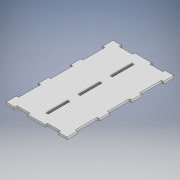
# Autodesk Inventor part: Lateral 1
Saved by Autodesk Inventor 2020 (Build 240168000, 168)
## iProperties
Created: 2020-03-11
Part Number: Lateral 1
Material: Generic
Document SubType Name: Modeling
Designer: José Javier Estrada
Density: 1 g/cm^3
Appearance: Default
Author: José Javier Estrada
Autodesk Inventor part; units mm, degrees
ref_plane "YZ Plane" through (0, 0, 0) normal (1, 0, 0) x (0, 1, 0)
ref_plane "XZ Plane" through (0, 0, 0) normal (0, 1, 0) x (-1, 0, 0)
ref_plane "XY Plane" through (0, 0, 0) normal (0, 0, 1) x (1, 0, 0)
sketch "Sketch1" plane through (0, 0, 0) normal (0, 1, 0) x (-1, 0, 0)
  line L0 (0, 0) -> (-140, 0)
  line L1 (-140, 0) -> (-140, 245)
  line L2 (-140, 245) -> (0, 245)
  line L3 (0, 245) -> (0, 0)
  dimension "d0" = 140
  dimension "d1" = 245
  constraints: 8 end point, 2 parallel, 1 horizontal, 1 perpendicular
  measures "d0" distance of L1.end L2.end
  measures "d1" distance of L0.end L1.end
extrude "Extrusion1" add sketch "Sketch1" along normal blind 5
sketch "Sketch2" plane through (0, 5, 0) normal (0, 1, 0) x (1, 0, 0)
  line L0 (0, -245) -> (140, -245) projected
  line L1 (140, -245) -> (140, 0) projected
  line L2 (140, 0) -> (0, 0) projected
  line L3 (0, 0) -> (0, -245) projected
  line L4 (135, -73.75) -> (140, -73.75)
  line L5 (140, -73.75) -> (140, -23.75)
  line L6 (140, -23.75) -> (135, -23.75)
  line L7 (135, -23.75) -> (135, -73.75)
  line L8 (135, -221.25) -> (140, -221.25)
  line L9 (140, -221.25) -> (140, -171.25)
  line L10 (140, -171.25) -> (135, -171.25)
  line L11 (135, -171.25) -> (135, -221.25)
  line L12 (135, -147.5) -> (140, -147.5)
  line L13 (140, -147.5) -> (140, -97.5)
  line L14 (140, -97.5) -> (135, -97.5)
  line L15 (135, -97.5) -> (135, -147.5)
  line L16 (0, -73.75) -> (5, -73.75)
  line L17 (5, -73.75) -> (5, -23.75)
  line L18 (5, -23.75) -> (0, -23.75)
  line L19 (0, -23.75) -> (0, -73.75)
  line L20 (0, -221.25) -> (5, -221.25)
  line L21 (5, -221.25) -> (5, -171.25)
  line L22 (5, -171.25) -> (0, -171.25)
  line L23 (0, -171.25) -> (0, -221.25)
  line L24 (0, -147.5) -> (5, -147.5)
  line L25 (5, -147.5) -> (5, -97.5)
  line L26 (5, -97.5) -> (0, -97.5)
  line L27 (0, -97.5) -> (0, -147.5)
  line L28 (20, -245) -> (50, -245)
  line L29 (50, -245) -> (50, -240)
  line L30 (50, -240) -> (20, -240)
  line L31 (20, -240) -> (20, -245)
  line L32 (90, -245) -> (120, -245)
  line L33 (120, -245) -> (120, -240)
  line L34 (120, -240) -> (90, -240)
  line L35 (90, -240) -> (90, -245)
  line L36 (20, -5) -> (50, -5)
  line L37 (50, -5) -> (50, 0)
  line L38 (50, 0) -> (20, 0)
  line L39 (20, 0) -> (20, -5)
  line L40 (120, 0) -> (90, 0)
  line L41 (90, 0) -> (90, -5)
  line L42 (90, -5) -> (120, -5)
  line L43 (120, -5) -> (120, 0)
  point P0 (140, -23.75)
  dimension "d4" = 50
  dimension "d5" = 5
  dimension "d6" = 50
  dimension "d7" = 5
  dimension "d8" = 50
  dimension "d9" = 5
  dimension "d10" = 23.75
  dimension "d11" = 23.75
  dimension "d12" = 23.75
  dimension "d13" = 50
  dimension "d14" = 5
  dimension "d15" = 50
  dimension "d16" = 5
  dimension "d17" = 50
  dimension "d18" = 5
  dimension "d19" = 23.75
  dimension "d20" = 23.75
  dimension "d21" = 23.75
  dimension "d22" = 20
  dimension "d23" = 5
  dimension "d25" = 30
  dimension "d26" = 5
  dimension "d27" = 30
  dimension "d28" = 5
  dimension "d29" = 30
  dimension "d30" = 5
  dimension "d31" = 30
  dimension "d32" = 20
  dimension "d33" = 20
  dimension "d34" = 20
  constraints: 80 end point, 20 parallel, 10 collinear, 10 horizontal, 10 perpendicular
  measures "d4" distance of L6.end L4.start
  measures "d5" distance of L5.end L6.end
  measures "d6" distance of L10.end L8.start
  measures "d7" distance of L9.end L10.end
  measures "d8" distance of L14.end L12.start
  measures "d9" distance of L13.end L14.end
  measures "d10" distance between parallel lines of L0 L8
  measures "d11" distance between parallel lines of L10 L12
  measures "d12" distance between parallel lines of L14 L4
  measures "d13" distance of L19.start L16.start
  measures "d14" distance of L17.end L19.start
  measures "d15" distance of L23.start L20.start
  measures "d16" distance of L21.end L23.start
  measures "d17" distance of L27.start L24.start
  measures "d18" distance of L25.end L27.start
  measures "d19" distance between parallel lines of L22 L24
  measures "d20" distance between parallel lines of L26 L16
  measures "d21" distance between parallel lines of L0 L20
  measures "d22" distance between parallel lines of L3 L31
  measures "d23" distance of L28.end L29.end
  measures "d25" distance of L28.start L28.end
  measures "d26" distance of L32.end L34.start
  measures "d27" distance of L35.end L32.end
  measures "d28" distance of L37.start L37.end
  measures "d29" distance of L36.start L37.start
  measures "d30" distance of L43.start L40.start
  measures "d31" distance of L41.end L43.start
  measures "d32" distance between parallel lines of L1 L33
  measures "d33" distance between parallel lines of L1 L43
  measures "d34" distance between parallel lines of L3 L39
extrude "Extrusion2" cut sketch "Sketch2" against normal blind 5 contours L31 L30 L29 L0 | L3 L22 L21 L20 | L35 L34 L33 L0 | L3 L26 L25 L24 | L3 L18 L17 L16 | L8 L11 L10 L1 | L12 L15 L14 L1 | L2 L37 L36 L39 | L4 L7 L6 L1 | L2 L43 L42 L41
sketch "Sketch3" plane through (0, 5, 0) normal (0, 1, 0) x (1, 0, 0)
  line L0 (0, -147.5) -> (5, -147.5) projected
  line L1 (5, -147.5) -> (5, -97.5) projected
  line L2 (5, -97.5) -> (0, -97.5) projected
  line L3 (0, -73.75) -> (0, -97.5) projected
  line L4 (0, -73.75) -> (5, -73.75) projected
  line L5 (5, -73.75) -> (5, -23.75) projected
  line L6 (5, -23.75) -> (0, -23.75) projected
  line L7 (0, 0) -> (0, -23.75) projected
  line L8 (20, 0) -> (0, 0) projected
  line L9 (20, 0) -> (20, -5) projected
  line L10 (20, -5) -> (50, -5) projected
  line L11 (50, -5) -> (50, 0) projected
  line L12 (90, 0) -> (50, 0) projected
  line L13 (90, 0) -> (90, -5) projected
  line L14 (90, -5) -> (120, -5) projected
  line L15 (120, -5) -> (120, 0) projected
  line L16 (140, 0) -> (120, 0) projected
  line L17 (140, -23.75) -> (140, 0) projected
  line L18 (140, -23.75) -> (135, -23.75) projected
  line L19 (135, -23.75) -> (135, -73.75) projected
  line L20 (135, -73.75) -> (140, -73.75) projected
  line L21 (140, -97.5) -> (140, -73.75) projected
  line L22 (140, -97.5) -> (135, -97.5) projected
  line L23 (135, -97.5) -> (135, -147.5) projected
  line L24 (135, -147.5) -> (140, -147.5) projected
  line L25 (140, -171.25) -> (140, -147.5) projected
  line L26 (140, -171.25) -> (135, -171.25) projected
  line L27 (135, -171.25) -> (135, -221.25) projected
  line L28 (135, -221.25) -> (140, -221.25) projected
  line L29 (140, -245) -> (140, -221.25) projected
  line L30 (120, -245) -> (140, -245) projected
  line L31 (120, -245) -> (120, -240) projected
  line L32 (120, -240) -> (90, -240) projected
  line L33 (90, -240) -> (90, -245) projected
  line L34 (50, -245) -> (90, -245) projected
  line L35 (50, -245) -> (50, -240) projected
  line L36 (50, -240) -> (20, -240) projected
  line L37 (20, -240) -> (20, -245) projected
  line L38 (0, -245) -> (20, -245) projected
  line L39 (0, -221.25) -> (0, -245) projected
  line L40 (0, -221.25) -> (5, -221.25) projected
  line L41 (5, -221.25) -> (5, -171.25) projected
  line L42 (5, -171.25) -> (0, -171.25) projected
  line L43 (0, -147.5) -> (0, -171.25) projected
  line L44 (135, -171.25) -> (135, -221.25) construction
  line L45 (135, -186.5648) -> (72.5, -186.5648) construction
  line L46 (67.5, -245) -> (72.5, -245)
  line L47 (72.5, 0) -> (67.5, 0)
  line L48 (67.5, -221.25) -> (72.5, -221.25)
  line L49 (67.5, -171.25) -> (72.5, -171.25)
  line L50 (67.5, -73.75) -> (72.5, -73.75)
  line L51 (67.5, -23.75) -> (72.5, -23.75)
  line L52 (67.5, -147.5) -> (72.5, -147.5)
  line L53 (67.5, -97.5) -> (72.5, -97.5)
  line L54 (67.5, -171.25) -> (67.5, -221.25)
  line L55 (72.5, -221.25) -> (72.5, -171.25)
  line L56 (72.5, -147.5) -> (72.5, -97.5)
  line L57 (72.5, -73.75) -> (72.5, -23.75)
  line L58 (67.5, -23.75) -> (67.5, -73.75)
  line L59 (67.5, -97.5) -> (67.5, -147.5)
  dimension "d37" = 62.5
  dimension "d39" = 23.75
  dimension "d40" = 50
  dimension "d41" = 23.75
  dimension "d42" = 50
  dimension "d43" = 50
  dimension "d44" = 23.75
  dimension "d45" = 5
  constraints: 30 end point, 12 parallel, 9 perpendicular, 6 collinear, 4 horizontal, 2 point on line
  measures "d37" distance of L45.start L45.end
  measures "d39" distance between parallel lines of L12 L51
  measures "d40" distance between parallel lines of L51 L50
  measures "d41" distance between parallel lines of L34 L48
  measures "d42" distance between parallel lines of L48 L49
  measures "d43" distance between parallel lines of L53 L52
  measures "d44" distance between parallel lines of L50 L53
  measures "d45" distance of L52.start L52.end
extrude "Extrusion3" cut sketch "Sketch3" against normal blind 5 contours L54 L49 L55 L48 | L58 L51 L57 L50 | L59 L53 L56 L52
body "Solid1"
